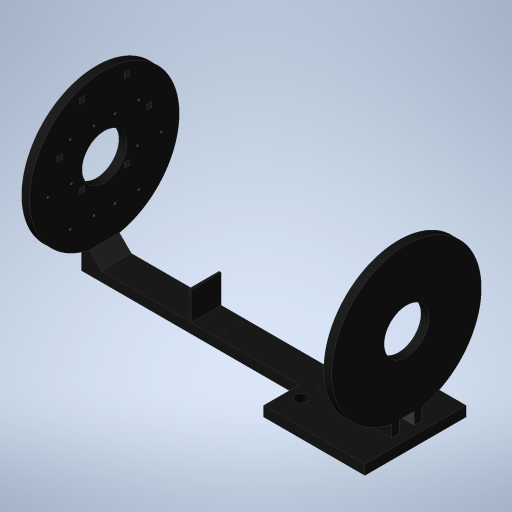
# Autodesk Inventor part: base2
Saved by Autodesk Inventor 2023 (Build 270158000, 158)
## iProperties
Created: 2022-11-02
Part Number: base2
Material: Generic
Document SubType Name: Modeling
Designer: Admin
Density: 1 g/cm^3
Appearance: Default
Author: Admin
Autodesk Inventor part; units mm, degrees
ref_plane "YZ Plane" through (0, 0, 0) normal (1, 0, 0) x (0, 1, 0)
ref_plane "XZ Plane" through (0, 0, 0) normal (0, 1, 0) x (-1, 0, 0)
ref_plane "XY Plane" through (0, 0, 0) normal (0, 0, 1) x (1, 0, 0)
sketch "Sketch1" plane through (0, 0, 0) normal (1, 0, 0) x (0, 1, 0)
  line L0 (38.9711, 22.5) -> (38.9711, -22.5)
  line L1 (0, -45) -> (-38.9711, -22.5)
  line L2 (-38.9711, -22.5) -> (-38.9711, 22.5)
  line L3 (-38.9711, 22.5) -> (0, 45)
  line L4 (0, 45) -> (38.9711, 22.5)
  line L5 (0, 45) -> (0, -45)
  line L6 (38.9711, 0) -> (-38.9711, 0)
  circle A0 centre (38.9711, -22.5) radius 17.5
  circle A1 centre (38.9711, -22.5) radius 15
  line L7 (38.9711, -22.5) -> (62.5188, -22.5)
  line L8 (56.4711, -26.5) -> (64.4711, -26.5)
  line L9 (64.4711, -26.5) -> (64.4711, -18.5)
  line L10 (64.4711, -18.5) -> (56.4711, -18.5)
  line L11 (56.4711, -18.5) -> (56.4711, -26.5)
  line L12 (56.4711, -26.5) -> (64.4711, -18.5) construction
  line L13 (64.4711, -26.5) -> (56.4711, -18.5) construction
  line L14 (38.9711, 22.5) -> (0, 0)
  line L15 (29.9645, 17.3) -> (28.1458, 16.25)
  line L16 (-48.9711, -15) -> (-48.9711, 15)
  line L17 (-48.9711, 15) -> (-56.9711, 15)
  line L18 (-56.9711, 15) -> (-56.9711, -15)
  line L19 (-56.9711, -15) -> (-48.9711, -15)
  circle A2 centre (-38.9711, -22.5) radius 17.5
  circle A3 centre (-38.9711, 22.5) radius 17.5
  line L20 (-52.9711, -15) -> (-52.9711, 15)
  line L21 (57.8711, -25.1) -> (63.0711, -25.1)
  line L22 (63.0711, -25.1) -> (63.0711, -19.9)
  line L23 (63.0711, -19.9) -> (57.8711, -19.9)
  line L24 (57.8711, -19.9) -> (57.8711, -25.1)
  line L25 (57.8711, -25.1) -> (63.0711, -19.9) construction
  line L26 (63.0711, -25.1) -> (57.8711, -19.9) construction
  circle A4 centre (38.9711, 22.5) radius 17.5
  circle A5 centre (0, 45) radius 17.5
  circle A6 centre (-38.9711, 22.5) radius 17.5
  circle A7 centre (-38.9711, -22.5) radius 17.5
  circle A8 centre (0, -45) radius 17.5
  line L27 (0, -45) -> (30.2711, -45)
  line L28 (17.5, -49) -> (25.5, -49)
  line L29 (25.5, -49) -> (25.5, -41)
  line L30 (25.5, -41) -> (17.5, -41)
  line L31 (17.5, -41) -> (17.5, -49)
  line L32 (17.5, -49) -> (25.5, -41) construction
  line L33 (25.5, -49) -> (17.5, -41) construction
  line L34 (18.9, -47.6) -> (24.1, -47.6)
  line L35 (24.1, -47.6) -> (24.1, -42.4)
  line L36 (24.1, -42.4) -> (18.9, -42.4)
  line L37 (18.9, -42.4) -> (18.9, -47.6)
  line L38 (18.9, -47.6) -> (24.1, -42.4) construction
  line L39 (24.1, -47.6) -> (18.9, -42.4) construction
  line L40 (-38.9711, -22.5) -> (-4.25, -22.5)
  line L41 (-21.4711, -26.5) -> (-13.4711, -26.5)
  line L42 (-13.4711, -26.5) -> (-13.4711, -18.5)
  line L43 (-13.4711, -18.5) -> (-21.4711, -18.5)
  line L44 (-21.4711, -18.5) -> (-21.4711, -26.5)
  line L45 (-21.4711, -26.5) -> (-13.4711, -18.5) construction
  line L46 (-13.4711, -26.5) -> (-21.4711, -18.5) construction
  line L47 (-20.0711, -25.1) -> (-14.8711, -25.1)
  line L48 (-14.8711, -25.1) -> (-14.8711, -19.9)
  line L49 (-14.8711, -19.9) -> (-20.0711, -19.9)
  line L50 (-20.0711, -19.9) -> (-20.0711, -25.1)
  line L51 (-20.0711, -25.1) -> (-14.8711, -19.9) construction
  line L52 (-14.8711, -25.1) -> (-20.0711, -19.9) construction
  line L53 (56.4711, 26.5) -> (64.4711, 26.5)
  line L54 (64.4711, 26.5) -> (64.4711, 18.5)
  line L55 (64.4711, 18.5) -> (56.4711, 18.5)
  line L56 (56.4711, 18.5) -> (56.4711, 26.5)
  line L57 (56.4711, 26.5) -> (64.4711, 18.5) construction
  line L58 (64.4711, 26.5) -> (56.4711, 18.5) construction
  line L59 (57.8711, 25.1) -> (63.0711, 25.1)
  line L60 (63.0711, 25.1) -> (63.0711, 19.9)
  line L61 (63.0711, 19.9) -> (57.8711, 19.9)
  line L62 (57.8711, 19.9) -> (57.8711, 25.1)
  line L63 (57.8711, 25.1) -> (63.0711, 19.9) construction
  line L64 (63.0711, 25.1) -> (57.8711, 19.9) construction
  line L65 (17.5, 49) -> (25.5, 49)
  line L66 (25.5, 49) -> (25.5, 41)
  line L67 (25.5, 41) -> (17.5, 41)
  line L68 (17.5, 41) -> (17.5, 49)
  line L69 (17.5, 49) -> (25.5, 41) construction
  line L70 (25.5, 49) -> (17.5, 41) construction
  line L71 (18.9, 47.6) -> (24.1, 47.6)
  line L72 (24.1, 47.6) -> (24.1, 42.4)
  line L73 (24.1, 42.4) -> (18.9, 42.4)
  line L74 (18.9, 42.4) -> (18.9, 47.6)
  line L75 (18.9, 47.6) -> (24.1, 42.4) construction
  line L76 (24.1, 47.6) -> (18.9, 42.4) construction
  line L77 (-21.4711, 26.5) -> (-13.4711, 26.5)
  line L78 (-13.4711, 26.5) -> (-13.4711, 18.5)
  line L79 (-13.4711, 18.5) -> (-21.4711, 18.5)
  line L80 (-21.4711, 18.5) -> (-21.4711, 26.5)
  line L81 (-21.4711, 26.5) -> (-13.4711, 18.5) construction
  line L82 (-13.4711, 26.5) -> (-21.4711, 18.5) construction
  line L83 (-20.0711, 25.1) -> (-14.8711, 25.1)
  line L84 (-14.8711, 25.1) -> (-14.8711, 19.9)
  line L85 (-14.8711, 19.9) -> (-20.0711, 19.9)
  line L86 (-20.0711, 19.9) -> (-20.0711, 25.1)
  line L87 (-20.0711, 25.1) -> (-14.8711, 19.9) construction
  line L88 (-14.8711, 25.1) -> (-20.0711, 19.9) construction
  line L89 (0, 0) -> (21.5, 0)
  circle A9 centre (21.5, 0) radius 55
  circle A10 centre (21.5, 0) radius 35
  line L90 (-31.415, 0) -> (-31.415, 15)
  line L91 (-31.415, 15) -> (-85.4711, 15)
  line L92 (-85.4711, 15) -> (-85.4711, 0)
  line L93 (-31.415, 7) -> (-85.4711, 7)
  line L94 (-85.4711, 15) -> (-95.4711, 15)
  line L95 (-95.4711, 15) -> (-95.4711, -10)
  line L96 (-31.415, 0) -> (-31.415, -15)
  line L97 (-31.415, -15) -> (-85.4711, -15)
  line L98 (-85.4711, -15) -> (-85.4711, 0)
  line L99 (-31.415, -7) -> (-85.4711, -7)
  line L100 (-85.4711, -15) -> (-95.4711, -15)
  line L101 (-95.4711, -15) -> (-95.4711, -10)
  circle A11 centre (38.9711, 22.5) radius 15
  circle A12 centre (0, 45) radius 15
  circle A13 centre (-38.9711, 22.5) radius 15
  circle A14 centre (-38.9711, -22.5) radius 15
  circle A15 centre (0, -45) radius 15
  line L102 (38.9711, -22.5) -> (30.2211, -7.3446)
  line L103 (0, -45) -> (-8.75, -29.8446)
  line L104 (-38.9711, -22.5) -> (-47.7211, -37.6554)
  circle A16 centre (0, 0) radius 22.5
  circle A17 centre (0, 0) radius 75
  circle A18 centre (38.9711, -22.5) radius 12.5
  circle A19 centre (32.0961, -10.5922) radius 1.05
  circle A20 centre (32.0961, -34.4078) radius 1.05
  circle A21 centre (38.9711, 22.5) radius 12.5
  circle A22 centre (0, 45) radius 12.5
  circle A23 centre (-38.9711, 22.5) radius 12.5
  circle A24 centre (-38.9711, -22.5) radius 12.5
  circle A25 centre (0, -45) radius 12.5
  circle A26 centre (-6.875, -33.0922) radius 1.05
  circle A27 centre (-6.875, -56.9078) radius 1.05
  circle A28 centre (-45.8461, -34.4078) radius 1.05
  circle A29 centre (-45.8461, -10.5922) radius 1.05
  circle A30 centre (32.0961, 10.5922) radius 1.05
  circle A31 centre (32.0961, 34.4078) radius 1.05
  circle A32 centre (-6.875, 33.0922) radius 1.05
  circle A33 centre (-6.875, 56.9078) radius 1.05
  circle A34 centre (-45.8461, 34.4078) radius 1.05
  circle A35 centre (-45.8461, 10.5922) radius 1.05
  point P0 (60.4711, -22.5)
  point P1 (21.5, -45)
  point P2 (-17.4711, -22.5)
  point P3 (60.4711, 22.5)
  point P4 (21.5, 45)
  point P5 (-17.4711, 22.5)
  point P6 (-31.415, -15)
  point P7 (-56.9711, 7)
  point P8 (-56.9711, -7)
  point P9 (-33.0527, 7)
  point P10 (-33.0527, -7)
  point P11 (-74.6726, 7)
  point P12 (-73.4847, 15)
  point P13 (-73.4847, -15)
  point P14 (-74.6726, -7)
  dimension "d8" = 35
  dimension "d45" = 110
  dimension "d9" = 45
  dimension "d12" = 30
  dimension "d13" = 8
  dimension "d14" = 8
  dimension "d22" = 30
  dimension "d23" = 8
  dimension "d24" = 30
  dimension "d25" = 35
  dimension "d26" = 35
  dimension "d27" = 4
  dimension "d30" = 5.2
  dimension "d31" = 5.2
  dimension "d34" = 360
  dimension "d36" = 8
  dimension "d37" = 8
  dimension "d38" = 5.2
  dimension "d39" = 5.2
  dimension "d40" = 8
  dimension "d41" = 8
  dimension "d42" = 5.2
  dimension "d43" = 5.2
  dimension "d44" = 21.5
  dimension "d46" = 70
  dimension "d47" = 15
  dimension "d49" = 8
  dimension "d50" = 28.5
  dimension "d51" = 10
  dimension "d97" = 360
  dimension "d99" = 120
  dimension "d102" = 120
  dimension "d105" = 120
  dimension "d112" = 45
  dimension "d113" = 150
  dimension "d118" = 25
  dimension "d119" = 18.5
  dimension "d120" = 2.1
  dimension "d122" = 13.75
  dimension "d125" = 360
  dimension "d127" = 2.1
  dimension "d128" = 13.75
  dimension "d129" = 2.1
  dimension "d130" = 13.75
  constraints: 210 end point, 41 symmetric about line, 32 centre point, 16 midpoint, 14 point on line, 12 horizontal, 11 parallel, 10 perpendicular, 7 coincident, 6 vertical, 1 tangent, 71 other
  measures "d9" distance of L0.start L0.end
  measures "d12" diameter of A1
  measures "d13" distance of L10.end L9.end
  measures "d14" distance of L8.end L9.end
  measures "d22" distance of L16.start L16.end
  measures "d23" distance of L17.start L17.end
  measures "d24" distance of L17.end L18.end
  measures "d25" diameter of A2
  measures "d26" diameter of A3
  measures "d27" distance between parallel lines of L18 L20
  measures "d30" distance of L23.end L22.end
  measures "d31" distance of L21.end L22.end
  measures "d36" distance of L30.end L29.end
  measures "d37" distance of L28.end L29.end
  measures "d38" distance of L36.end L35.end
  measures "d39" distance of L34.end L35.end
  measures "d40" distance of L43.end L42.end
  measures "d41" distance of L41.end L42.end
  measures "d42" distance of L49.end L48.end
  measures "d43" distance of L47.end L48.end
  measures "d44" distance of L14.end L89.end
  measures "d46" diameter of A10
  measures "d47" distance of L90.start L90.end
  measures "d49" distance between parallel lines of L91 L93
  measures "d50" distance between parallel lines of L18 L92
  measures "d51" distance of L91.end L94.end
  measures "d99" angle of L7 L102
  measures "d102" angle of L27 L103
  measures "d105" angle of L40 L104
  measures "d112" diameter of A16
  measures "d113" diameter of A17
  measures "d118" diameter of A18
  measures "d119" distance between parallel lines of L89 L10
  measures "d120" diameter of A19
  measures "d122" distance of A19.centre L0.end
  measures "d127" diameter of A26
  measures "d128" distance of L27.start A26.centre
  measures "d129" diameter of A28
  measures "d130" distance of L1.end A28.centre
extrude "Extrusion1" add sketch "Sketch1" along normal blind 8 contours L4 A21 A10 L0 | L14 A21 L4 | L0 A21 L14 | A21 A10 A11 L0 | L0 A11 L14 A21 | A21 L14 A11 L4 | L4 A11 A10 A31 A21 | A11 A10 A4 L0 | L0 A4 L14 A11 | A21 A10 A31 A11 | A10 A21 | A11 L14 A4 L4 | L4 A4 A10 A11 | A4 A10 A0 L0 | L0 L6 A16 L14 A4 | A11 A10 A4 | A4 L14 A16 L5 A5 A10 L4 | L4 A10 A4 | A31 A10 | A10 A31 | L0 A0 A10 A8 L5 A16 L6 | L11 L10 L9 L8 | L31 L30 L29 L27 L35 L36 L37 | L27 L37 L34 L35 L29 L28 L31 | L68 L65 L66 L67 | L56 L53 L54 L55 | A4 A10 L4 A5 A9 A17 A8 A0 | A10 A5 L4 | A0 A10 A1 L0 | L0 A1 L102 A0 | A16 L5 L6 | L6 L14 A16 | L14 L5 A16 | A5 A10 A12 L4 | L4 A12 A9 A5 | A5 L5 A10 A12 | A1 A10 A18 L0 | L0 A18 L102 A19 A1 | A0 L7 A1 A10 | L102 A1 A10 A0 | A16 A10 L6 L5 | L5 A8 A10 A16 | L6 A10 A16 L5 | A16 A10 A5 L5 | A12 A10 L5 A22 L4 | L4 A22 A9 A12 | A5 A10 L5 | A12 A10 | A18 A10 L7 L0 | L0 L102 A18 | A1 L7 A18 A10 | L102 A19 A18 A10 A20 A1 | A0 A10 A1 L7 | A8 A10 A15 L5 | L5 A10 A8 | A16 L6 A10 | A10 L40 L42 L43 L44 A2 L96 L6 A16 | L6 A16 A10 | L80 L77 L78 L79 | A16 L6 L90 A3 A9 L3 A5 A10 | A22 L5 L4 | L4 L3 A22 A9 | A9 A12 A5 | A5 A9 L3 A3 L17 L91 A17 | A10 A5 L3 A12 L5 | L5 A12 A10 | L7 A10 A18 L102 | A18 L7 A10 | A1 A10 A20 A18 L7 | A19 L102 | L102 A19 | A8 L27 A15 A10 | A10 A15 L5 | L5 A15 L103 A8 A10 | A8 L1 A9 A2 L44 L41 L42 L40 A10 | L5 A22 L3 | L5 A12 L3 A22 | A9 A22 A12 | A9 A12 L3 A5 | A5 L3 A9 | L7 A18 A10 | A20 A10 | A10 A20 | A8 A9 A15 L27 | A15 L27 A25 L5 A10 | A10 A15 | L5 A25 L103 A26 A15 | L103 A15 L1 A8 | L42 L41 L44 L40 L50 L47 L48 | L40 L48 L49 L50 L44 L43 L42 | L96 A2 A9 L6 | L6 A9 A3 L90 | L3 A12 A9 A22 | A9 A22 | A9 A3 L3 | A17 L93 L92 L91 | L91 L18 L93 A17 | A9 A17 L97 L19 A2 L1 A8 | A8 A9 A15 | A15 A9 A25 L27 | L37 L36 L35 L27 | L27 L35 L34 L37 | A25 L27 L5 | L5 L103 A25 | L103 A26 A25 L1 A15 | A8 A9 L1 | L1 A15 A9 A8 | L48 L47 L50 L40 | L40 L50 L49 L48 | A9 A2 L2 L6 | L6 L2 A3 A9 | L90 A13 A9 A3 | A3 A9 L93 L90 | L96 L99 A9 A2 | A2 L40 A14 L96 | A3 A9 A13 L3 | L3 A13 L17 A3 | L17 A3 L20 L93 L18 | L92 L98 L100 L101 L95 L94 | A17 L99 L98 L92 L93 | L93 L18 L99 A17 | A15 A9 A25 | A25 A9 L1 L27 | L1 A25 L103 | L1 A25 A9 A15 | A26 L103 | L103 A26 | L1 A2 A9 | L2 A2 L99 L16 L93 A3 | A3 L2 L93 A9 | A9 L99 L2 A2 | L93 A9 A13 L90 | A2 A9 A14 L40 | L96 A14 A9 L99 | A13 A9 A23 L3 | L3 A23 L17 A13 | L17 L20 A3 | A13 L90 A23 A9 | A17 L99 L18 L97 | L97 L98 L99 A17 | L93 L20 L99 L18 | A25 A9 | A2 L104 A14 L1 | L1 A14 A9 A2 | L2 L99 A2 | A3 L93 L2 | L93 L2 A13 A9 | A9 A14 L2 L99 | A13 A9 A23 L90 | A14 A9 A24 L40 | L40 A24 L96 A14 | L96 A24 A9 A14 | A23 A9 L91 L2 L3 | L3 L2 L91 A23 | A13 L16 A3 L20 L17 | L17 L16 A13 | A3 L16 L93 L20 | A23 L90 A9 | L18 L99 L20 A2 L19 | L93 L16 L99 L20 | A14 L104 A28 A24 L1 | L1 A24 A9 A14 | A2 L19 A14 L104 | L2 A14 L16 A2 L99 | A2 L16 L99 | L93 A3 L16 A13 L2 | L93 L16 A3 | A13 L2 A23 A9 | A9 A24 L2 A14 | A23 A9 L90 | A24 A9 L40 | L40 A9 L96 A24 | L96 A9 A24 | A23 L2 A13 L16 | L91 L2 A23 | A9 A23 L2 L91 | A2 L20 L19 | L99 L16 A2 L20 | A24 L104 L1 | L1 L40 A9 A24 | A14 L19 A24 L104 A28 | L2 A24 L16 A14 | L16 A14 L19 L20 A2 | A9 L97 L2 A24 | L40 L2 L97 A9 | L104 A24 L97 L2 | A14 L16 L19 | A28 L104 | L104 A28 | L2 L97 A24 | L24 L23 L22 L21 | L59 L60 L61 L62 | L71 L72 L73 L74 | L83 L84 L85 L86 | A27 | A29 | A30 | A32 | A33 | A34 | A35
extrude "Extrusion2" cut sketch "Sketch1" along normal blind 10 contours A16 L5 L6 | L6 L14 A16 | L14 L5 A16 | A16 A10 L6 L5 | L6 A10 A16 L5 | A16 L6 A10 | L6 A16 A10 | L37 L36 L35 L27 | L27 L35 L34 L37 | L48 L47 L50 L40 | L40 L50 L49 L48 | L24 L23 L22 L21 | L59 L60 L61 L62 | L71 L72 L73 L74 | L83 L84 L85 L86
extrude "Extrusion3" add sketch "Sketch1" along normal blind 320 contours L92 L98 L100 L101 L95 L94
sketch "Sketch2" plane through (0, -95.4711, -15) normal (0, -1, 0) x (1, 0, 0)
  line L0 (320, 0) -> (320, 30) projected
  line L1 (320, 15) -> (239.7614, 15)
  line L2 (218.4, -35.8) -> (320, -35.8)
  line L3 (320, -35.8) -> (320, 65.8)
  line L4 (320, 65.8) -> (218.4, 65.8)
  line L5 (218.4, 65.8) -> (218.4, -35.8)
  line L6 (218.4, -35.8) -> (320, 65.8) construction
  line L7 (320, -35.8) -> (218.4, 65.8) construction
  line L8 (320, 30) -> (320, 0) projected
  circle A0 centre (231.1, -10.4) radius 6
  circle A1 centre (294.9, 15) radius 3.25
  line L9 (8, -40) -> (8, 70) projected
  line L10 (8, 50) -> (8, -20) projected
  line L11 (8, 15) -> (110, 15)
  line L12 (110, 15) -> (135.5, 15)
  line L13 (135.5, 15) -> (135.5, 6.5)
  circle A2 centre (135.5, 6.5) radius 1.5
  circle A3 centre (135.5, 23.5) radius 1.5
  circle A4 centre (230.5, 6.5) radius 1.5
  circle A5 centre (230.5, 23.5) radius 1.5
  circle A6 centre (231.1, 40.4) radius 6
  line L14 (110, 0) -> (108, 0)
  line L15 (108, 0) -> (108, 30)
  line L16 (108, 30) -> (110, 30)
  line L17 (110, 30) -> (110, 0)
  line L18 (8, -60) -> (8, 90) projected
  line L19 (0, -60) -> (0, 90) projected
  point P0 (0, 15)
  point P1 (269.2, 15)
  point P2 (8, 0)
  point P3 (8, 30)
  point P4 (0, 0)
  point P5 (0, 30)
  dimension "d58" = 101.6
  dimension "d59" = 101.6
  dimension "d60" = 12
  dimension "d63" = 6.5
  dimension "d65" = 102
  dimension "d66" = 25.5
  dimension "d67" = 8.5
  dimension "d68" = 3
  dimension "d71" = 95
  dimension "d80" = 25.4
  dimension "d81" = 12.7
  dimension "d82" = 76.5
  dimension "d92" = 2
  dimension "d131" = 2
  constraints: 28 end point, 7 centre point, 6 horizontal, 5 midpoint, 4 parallel, 3 perpendicular, 2 point on line, 2 symmetric about line, 1 coincident, 1 collinear, 7 other
  measures "d58" distance of L4.end L3.end
  measures "d59" distance of L2.end L3.end
  measures "d60" diameter of A0
  measures "d63" diameter of A1
  measures "d65" distance of L11.start L11.end
  measures "d66" distance of L11.end L12.end
  measures "d67" distance of L12.end L13.end
  measures "d68" diameter of A2
  measures "d71" distance of A2.centre A4.centre
  measures "d80" distance from line of L2 A0.centre
  measures "d81" distance from line of L5 A0.centre
  measures "d82" distance from line of L5 A1.centre
  measures "d92" distance between parallel lines of L15 L17
  measures "d131" distance from line of L15 L11.end
extrude "Extrusion4" add sketch "Sketch2" against normal blind 10 contours L3 L2 L5 L4 L0
extrude "Extrusion5" cut sketch "Sketch2" against normal blind 10 contours A2 | A3 | A4 | A5
pattern_linear "Rectangular Pattern1" count 2 spacing 303 along (1, 0, 0) of "Extrusion1", "Extrusion2"
sketch "Sketch3" plane through (0, 0, 0) normal (-1, 0, 0) x (0, 0, 1)
  line L0 (-25.1, -20.0711) -> (-25.1, -14.8711) projected
  line L1 (-25.1, -14.8711) -> (-19.9, -14.8711) projected
  line L2 (-19.9, -14.8711) -> (-19.9, -20.0711) projected
  line L3 (-19.9, -20.0711) -> (-25.1, -20.0711) projected
  line L4 (-42.4, 24.1) -> (-42.4, 18.9) projected
  line L5 (-42.4, 18.9) -> (-47.6, 18.9) projected
  line L6 (-47.6, 18.9) -> (-47.6, 24.1) projected
  line L7 (-47.6, 24.1) -> (-42.4, 24.1) projected
  line L8 (25.1, 63.0711) -> (25.1, 57.8711) projected
  line L9 (25.1, 57.8711) -> (19.9, 57.8711) projected
  line L10 (19.9, 57.8711) -> (19.9, 63.0711) projected
  line L11 (19.9, 63.0711) -> (25.1, 63.0711) projected
  line L12 (25.1, -20.0711) -> (19.9, -20.0711) projected
  line L13 (19.9, -20.0711) -> (19.9, -14.8711) projected
  line L14 (19.9, -14.8711) -> (25.1, -14.8711) projected
  line L15 (25.1, -14.8711) -> (25.1, -20.0711) projected
  line L16 (-19.9, 63.0711) -> (-19.9, 57.8711) projected
  line L17 (-19.9, 57.8711) -> (-25.1, 57.8711) projected
  line L18 (-25.1, 57.8711) -> (-25.1, 63.0711) projected
  line L19 (-25.1, 63.0711) -> (-19.9, 63.0711) projected
  line L20 (47.6, 18.9) -> (42.4, 18.9) projected
  line L21 (42.4, 18.9) -> (42.4, 24.1) projected
  line L22 (42.4, 24.1) -> (47.6, 24.1) projected
  line L23 (47.6, 24.1) -> (47.6, 18.9) projected
  point P0 (0, 0)
extrude "Extrusion7" add sketch "Sketch3" against normal blind 3.1
sketch "Sketch4" plane through (311, -85.4711, -15) normal (1, 0, 0) x (0, 0, -1)
  line L0 (-57.4, 104.3711) -> (-62.6, 104.3711) projected
  line L1 (-62.6, 104.3711) -> (-62.6, 109.5711) projected
  line L2 (-62.6, 109.5711) -> (-57.4, 109.5711) projected
  line L3 (-57.4, 109.5711) -> (-57.4, 104.3711) projected
  line L4 (4.9, 143.3423) -> (4.9, 148.5423) projected
  line L5 (4.9, 148.5423) -> (10.1, 148.5423) projected
  line L6 (10.1, 148.5423) -> (10.1, 143.3423) projected
  line L7 (10.1, 143.3423) -> (4.9, 143.3423) projected
  line L8 (-34.9, 65.4) -> (-40.1, 65.4) projected
  line L9 (-40.1, 65.4) -> (-40.1, 70.6) projected
  line L10 (-40.1, 70.6) -> (-34.9, 70.6) projected
  line L11 (-34.9, 70.6) -> (-34.9, 65.4) projected
  line L12 (-40.1, 143.3423) -> (-40.1, 148.5423) projected
  line L13 (-40.1, 148.5423) -> (-34.9, 148.5423) projected
  line L14 (-34.9, 148.5423) -> (-34.9, 143.3423) projected
  line L15 (-34.9, 143.3423) -> (-40.1, 143.3423) projected
  line L16 (27.4, 104.3711) -> (27.4, 109.5711) projected
  line L17 (27.4, 109.5711) -> (32.6, 109.5711) projected
  line L18 (32.6, 109.5711) -> (32.6, 104.3711) projected
  line L19 (32.6, 104.3711) -> (27.4, 104.3711) projected
  line L20 (10.1, 70.6) -> (10.1, 65.4) projected
  line L21 (10.1, 65.4) -> (4.9, 65.4) projected
  line L22 (4.9, 65.4) -> (4.9, 70.6) projected
  line L23 (4.9, 70.6) -> (10.1, 70.6) projected
  line L24 (0, 0) -> (-30, 0) projected
  line L25 (0, 0) -> (0, 11.9865) projected
  arc A0 (0, 11.9865) -> (-30, 11.9865) centre (-15, 85.4711) ccw projected
  line L26 (-30, 11.9865) -> (-30, 0) projected
extrude "Extrusion8" add sketch "Sketch4" against normal blind 3.1 contours L0 L1 L2 L3 | L4 L5 L6 L7 | L8 L9 L10 L11 | L12 L13 L14 L15 | L16 L17 L18 L19 | L20 L21 L22 L23
extrude "Extrusion9" add sketch "Sketch2" against normal blind 38.5 contours L15 L16 L17 L11 | L11 L17 L14 L15
sketch "Sketch7" plane through (0, 0, 0) normal (-1, 0, 0) x (0, 0, 1)
  circle A0 centre (0, 0) radius 22.5
  circle A1 centre (0, 0) radius 75
  dimension "d108" = 45
  dimension "d109" = 150
  constraints: 2 centre point, 2 coincident
  measures "d108" diameter of A0
  measures "d109" diameter of A1
extrude "Extrusion11" cut sketch "Sketch1" along normal blind 10 contours A31 A10 | A10 A31 | A19 L102 | L102 A19 | A20 A10 | A10 A20 | A26 L103 | L103 A26 | A28 L104 | L104 A28 | A27 | A29 | A30 | A32 | A33 | A34 | A35
extrude "Extrusion12" add sketch "Sketch1" along normal blind 6.9 contours A31 A10 | A10 A31 | A19 L102 | L102 A19 | A20 A10 | A10 A20 | A26 L103 | L103 A26 | A28 L104 | L104 A28 | A27 | A29 | A30 | A32 | A33 | A34 | A35
sketch "Sketch8" plane through (0, -95.4711, -15) normal (0, 0, -1) x (-1, 0, 0)
  line L0 (-8, 10) -> (-8, 21.9865) projected
  line L1 (-8, 21.9865) -> (-20.1402, 9.8463)
  line L2 (-303, 10) -> (-303, 21.9865) projected
  line L3 (-303, 21.9865) -> (-291.0135, 10)
  line L4 (-8, 10) -> (-108, 10) projected
  line L5 (-320, 10) -> (-218.4, 10) projected
  line L6 (-303, 10) -> (-291.0135, 10)
  point P0 (0, 95.4711)
  point P1 (-19.9865, 10)
  dimension "d132" = 45
  dimension "d133" = 45
  constraints: 6 end point, 1 horizontal
  measures "d132" angle of L0 L1
  measures "d133" angle of L2 L3
extrude "Extrusion13" add sketch "Sketch8" against normal blind 30
sketch "Sketch9" plane through (311, -85.4711, -15) normal (1, 0, 0) x (0, 0, -1)
  line L0 (0, 11.9865) -> (-30, 11.9865) projected
  line L1 (-30, 11.9865) -> (-30, 0) projected
  line L2 (0, 0) -> (0, 11.9865) projected
  line L3 (-65.8, 0) -> (35.8, 0) projected
  line L4 (-22.5, 11.9865) -> (-22.5, 0)
  line L5 (-30, 0) -> (0, 0) projected
  line L6 (-7.5, 0) -> (-7.5, 11.9865)
  point P0 (-15, 85.4711)
  point P1 (-22.5, 5.9932)
  point P2 (-7.5, 0)
  dimension "d136" = 7.5
  dimension "d137" = 7.5
  constraints: 4 end point, 4 point on line, 1 midpoint, 1 parallel, 1 vertical
  measures "d136" distance from line of L1 point (-22.5, 5.993)
  measures "d137" distance between parallel lines of L2 L6
extrude "Extrusion14" cut sketch "Sketch9" against normal blind 30 contours L6 L3 L4 L0
equation "\"d14\" = d13"
equation "\"d31\" = d30"
equation "\"d37\" = d36"
equation "\"d39\" = d38"
equation "\"d41\" = d40"
equation "\"d43\" = d42"
body "Solid1"
